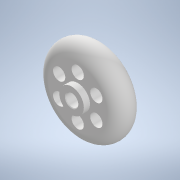
# Autodesk Inventor part: Koło
Saved by Autodesk Inventor 2021 (Build 250183000, 183)
## iProperties
Created: 2021-05-12
Part Number: Koło
Material: Ogólny
Document SubType Name: Modeling
Designer: DESKTOP-12
Density: 1 g/cm^3
Appearance: Domyślna
Author: DESKTOP-12
Autodesk Inventor part; units mm, degrees
ref_plane "YZ Plane" through (0, 0, 0) normal (1, 0, 0) x (0, 1, 0)
ref_plane "XZ Plane" through (0, 0, 0) normal (0, 1, 0) x (-1, 0, 0)
ref_plane "XY Plane" through (0, 0, 0) normal (0, 0, 1) x (1, 0, 0)
sketch "Szkic1" plane through (0, 0, 0) normal (0, 1, 0) x (-1, 0, 0)
  line L0 (0, 0) -> (0, 15)
  line L1 (0, 15) -> (10, 15)
  line L2 (10, 15) -> (10, 10)
  line L3 (10, 10) -> (34, 10)
  line L4 (34, 10) -> (34, -10)
  line L5 (34, -10) -> (10, -10)
  line L6 (10, -10) -> (10, -15)
  line L7 (10, -15) -> (0, -15)
  line L8 (0, -15) -> (0, 0)
  dimension "d0" = 15
  dimension "d1" = 10
  dimension "d2" = 5
  dimension "d3" = 24
  dimension "d4" = 20
  dimension "d5" = 24
  dimension "d6" = 5
  constraints: 18 end point, 6 perpendicular, 3 point on line, 1 vertical
  measures "d0" distance of L0.start L0.end
  measures "d1" distance of L0.end L1.end
  measures "d2" distance of L1.end L2.end
  measures "d3" distance of L2.end L3.end
  measures "d4" distance of L3.end L4.end
  measures "d5" distance of L4.end L5.end
  measures "d6" distance of L5.end L6.end
revolve "Obrót1" add sketch "Szkic1" angle 360 about axis through (0, 0, -15) along (0, 0, 1)
fillet "Zaokrąglenie1" radius 10 2 edges at (34, 0, 10) (34, 0, -10)
sketch "Szkic2" plane through (0, 0, 15) normal (0, 0, 1) x (1, 0, 0)
  point P0 (0, 0)
  point P1 (0, 0)
  constraints: 1 coincident
hole "Otwór1" at (0, 0, 15) direction (0, 0, -1) diameter 10 end through all
sketch "Szkic3" plane through (0, 0, 10) normal (0, 0, 1) x (1, 0, 0)
  circle A0 centre (0, 0) radius 17.5
  circle A1 centre (0, 17.5) radius 5
  dimension "d16" = 35
  dimension "d17" = 10
  constraints: 1 centre point, 1 coincident, 1 vertical alignment, 2 other
  measures "d17" diameter of A1
extrude "Wyciągnięcie proste1" cut sketch "Szkic3" against normal through all contours A1 A0 | A0 A1 picked at (0, 15.7801) picked at (-0.1194, 19.1092)
chamfer "Faza1" distance 0.5 angle 45 2 edges at (0, 5, 15) (0, 5, -15)
pattern_circular "Szyk kołowy1" count 6 over 360 about axis through (0, 0, 12.5) along (0, 0, -1) of "Wyciągnięcie proste1"
